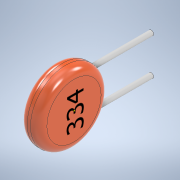
# Autodesk Inventor part: cap334
Saved by Autodesk Inventor 2020 (Build 240168000, 168)
## iProperties
Created: 2021-10-19
Part Number: cap334
Material: Genérico
Document SubType Name: Modeling
Designer: DANIEL
Density: 1 g/cm^3
Appearance: Valor por defecto
Author: DANIEL
Autodesk Inventor part; units mm, degrees
ref_plane "YZ Plane" through (0, 0, 0) normal (1, 0, 0) x (0, 1, 0)
ref_plane "XZ Plane" through (0, 0, 0) normal (0, 1, 0) x (-1, 0, 0)
sketch "Boceto1" plane through (0, 0, 0) normal (1, 0, 0) x (0, 1, 0)
  circle A0 centre (0, 0) radius 2.15
  dimension "d0" = 4.3
  constraints: 1 centre point, 1 coincident
  measures "d0" diameter of A0
extrude "Extrusión1" add sketch "Boceto1" along normal mid plane 1.2
fillet "Empalme1" radius 0.5 1 edges at (0.6, -2.15, 0)
fillet "Empalme2" radius 0.5 1 edges at (-0.6, -2.15, 0)
sketch "Boceto2" plane through (-0.6, 0, 0) normal (-1, 0, 0) x (0, 0, 1)
  line L0 (0.4589, 1.19) -> (0.433, -1.0611) construction
  line L1 (0.433, -1.0611) -> (-0.6091, -1.0491) construction
  line L2 (-0.6091, -1.0491) -> (-0.5832, 1.202) construction
  line L3 (-0.5832, 1.202) -> (0.4589, 1.19) construction
  point P0 (0, 0)
  constraints: 2 other
sketch "Boceto3" plane through (0.6, 0, 0) normal (1, 0, 0) x (0, 0, -1)
  line L0 (-0.4506, -1.1931) -> (-0.4404, 1.0581) construction
  line L1 (-0.4404, 1.0581) -> (0.6018, 1.0533) construction
  line L2 (0.6018, 1.0533) -> (0.5916, -1.1979) construction
  line L3 (0.5916, -1.1979) -> (-0.4506, -1.1931) construction
  point P0 (0, 0)
  constraints: 2 other
ref_plane "Plano de trabajo1" through (0, 0, -1.3) normal (0, 0, 1) x (1, 0, 0)
sketch "Boceto4" plane through (0, 0, -1.3) normal (0, 0, 1) x (1, 0, 0)
  line L0 (0.1, -2.15) -> (0.1, 2.15) projected
  line L1 (0.6, 1.65) -> (0.6, -1.65) projected
  line L2 (-0.1, 2.15) -> (-0.1, -2.15) projected
  line L3 (-0.6, -1.65) -> (-0.6, 1.65) projected
  line L4 (0.1, -2.15) -> (0.1, 2.15) projected
  line L5 (-0.1, 2.15) -> (-0.1, -2.15) projected
  circle A0 centre (0, -1.0922) radius 0.15
  circle A1 centre (0, 1.152) radius 0.15
  point P0 (0, 0)
  dimension "d7" = 0.3
  dimension "d8" = 0.3
  constraints: 2 centre point
  measures "d7" diameter of A0
  measures "d8" diameter of A1
extrude "Extrusión2" add sketch "Boceto4" against normal blind 4 contours A0 L2 L0 | L0 A0 | A0 L2 | A1 L2 L0 | L0 A1 | A1 L2
